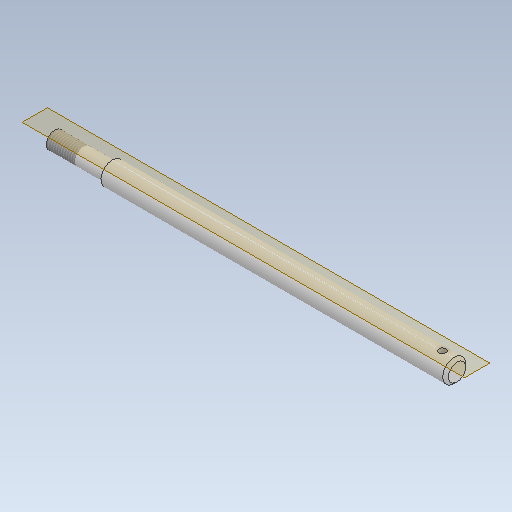
# Autodesk Inventor part: Part7
Saved by Autodesk Inventor 2021 (Build 250183000, 183)
## iProperties
Created: 2022-06-05
Part Number: Part7
Material: Generic
Document SubType Name: Modeling
Designer: Bhargav Malasani
Density: 1 g/cm^3
Appearance: Default
Author: Bhargav Malasani
Autodesk Inventor part; units mm, degrees
ref_plane "YZ Plane" through (0, 0, 0) normal (1, 0, 0) x (0, 1, 0)
ref_plane "XY Plane" through (0, 0, 0) normal (0, 0, 1) x (1, 0, 0)
sketch "Sketch1" plane through (0, 0, 0) normal (0, 0, 1) x (1, 0, 0)
  line L0 (0, 0) -> (280, 0)
  line L1 (280, 0) -> (280, 6)
  line L2 (0, 0) -> (0, 6)
  line L3 (0, 6) -> (40, 6)
  line L4 (40, 6) -> (40, 8)
  line L5 (40, 8) -> (278, 8)
  line L6 (278, 8) -> (280, 6)
  point P0 (280, 8)
  dimension "d0" = 280
  dimension "d1" = 8
  dimension "d2" = 6
  dimension "d3" = 40
  dimension "d4" = 2
  dimension "d5" = 2
  dimension "d6" = 45
  constraints: 14 end point, 2 perpendicular, 2 point on line, 2 vertical, 1 horizontal
  measures "d0" distance of L0.start L0.end
  measures "d1" distance of L0.end point (280, 8)
  measures "d2" distance of L0.start L2.end
  measures "d3" distance of L2.end L3.end
  measures "d4" distance of L3.end L4.end
  measures "d5" distance of L5.end point (280, 8)
  measures "d6" angle of L5 L6
revolve "Revolution1" add sketch "Sketch1" angle 360 about axis through (0, 0, 0) along (1, 0, 0)
thread "Thread1" size "M12x1.75" class "6g" standard "ANSI Metric M Profile" length 20
ref_plane "Work Plane1" through (0, 8, 0) normal (0, 1, 0) x (-1, 0, 0)
sketch "Sketch2" plane through (0, 8, 0) normal (0, 1, 0) x (-1, 0, 0)
  circle A0 centre (-270, 0) radius 2.5
  line L0 (-280, 6) -> (-280, -6) projected
  point P0 (0, 0)
  dimension "d12" = 5
  dimension "d13" = 10
  dimension "d14" = 270
  constraints: 1 centre point
  measures "d12" diameter of A0
  measures "d13" distance from line of L0 A0.centre
  measures "d14" distance of A0.centre point (0, 0)
extrude "Extrusion1" cut sketch "Sketch2" against normal through all
body "Solid1"
